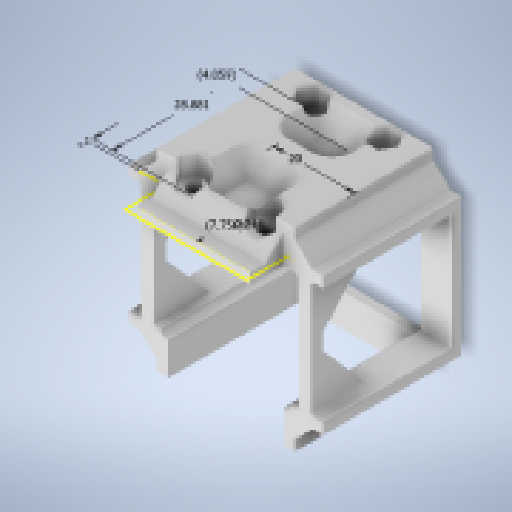
# Autodesk Inventor part: 56-spiralxy-groove-FocusToCubeAdapter
Saved by Autodesk Inventor 2024.1 (Build 281209000, 209)
## iProperties
Created: 2023-11-15
Part Number: 56-spiralxy-groove-FocusToCubeAdapter
Material: Generisch
Document SubType Name: Modeling
Designer: buchmannmartin
Density: 1 g/cm^3
Appearance: Vorgabe
Author: buchmannmartin
Autodesk Inventor part; units mm, degrees
ref_plane "YZ Plane" through (0, 0, 0) normal (1, 0, 0) x (0, 1, 0)
ref_plane "XZ Plane" through (0, 0, 0) normal (0, 1, 0) x (-1, 0, 0)
ref_plane "XY Plane" through (0, 0, 0) normal (0, 0, 1) x (1, 0, 0)
sketch "Skizze1" plane through (0, 0, 0) normal (0, 0, 1) x (1, 0, 0)
  line L0 (17.02, 23.9) -> (17.02, 21.2698) construction
  line L1 (17.02, 21.2698) -> (21.2698, 17.02) construction
  line L2 (21.2698, 17.02) -> (23.9, 17.02) construction
  line L3 (-23.9, 17.02) -> (-21.2698, 17.02) construction
  line L4 (-21.2698, 17.02) -> (-17.02, 21.2698) construction
  line L5 (-17.02, 21.2698) -> (-17.02, 23.9) construction
  line L6 (-17.02, -23.9) -> (-17.02, -21.2698) construction
  line L7 (-17.02, -21.2698) -> (-21.2698, -17.02) construction
  line L8 (-21.2698, -17.02) -> (-23.9, -17.02) construction
  line L9 (23.9, -17.02) -> (21.2698, -17.02) construction
  line L10 (21.2698, -17.02) -> (17.02, -21.2698) construction
  line L11 (17.02, -21.2698) -> (17.02, -23.9) construction
  line L12 (-14.5, 14.25) -> (14.5, 14.25)
  line L13 (16, 12.75) -> (16, -14.25)
  line L14 (14.5, -15.75) -> (-14.5, -15.75)
  line L15 (-16, -14.25) -> (-16, 12.75)
  line L16 (17.02, 23.9) -> (-17.02, 23.9) construction
  line L17 (-23.9, 17.02) -> (-23.9, -17.02) construction
  line L18 (23.9, -17.02) -> (23.9, 17.02) construction
  line L19 (17.02, -23.9) -> (-17.02, -23.9) construction
  line L20 (-16.92, 23.8) -> (-16.92, 21.2284)
  line L21 (-16.92, 21.2284) -> (-21.2284, 16.92)
  line L22 (-21.2284, 16.92) -> (-23.8, 16.92)
  line L23 (-23.8, 16.92) -> (-23.8, -16.92)
  line L24 (-23.8, -16.92) -> (-21.2284, -16.92)
  line L25 (-21.2284, -16.92) -> (-16.92, -21.2284)
  line L26 (-16.92, -21.2284) -> (-16.92, -23.8)
  line L27 (-16.92, -23.8) -> (16.92, -23.8)
  line L28 (16.92, -23.8) -> (16.92, -21.2284)
  line L29 (16.92, -21.2284) -> (21.2284, -16.92)
  line L30 (21.2284, -16.92) -> (23.8, -16.92)
  line L31 (23.8, -16.92) -> (23.8, 16.92)
  line L32 (23.8, 16.92) -> (21.2284, 16.92)
  line L33 (21.2284, 16.92) -> (16.92, 21.2284)
  line L34 (16.92, 21.2284) -> (16.92, 23.8)
  line L35 (16.92, 23.8) -> (-16.92, 23.8)
  arc A0 (16, 12.75) -> (14.5, 14.25) centre (14.5, 12.75) ccw
  arc A1 (14.5, -15.75) -> (16, -14.25) centre (14.5, -14.25) ccw
  arc A2 (-16, -14.25) -> (-14.5, -15.75) centre (-14.5, -14.25) ccw
  arc A3 (-14.5, 14.25) -> (-16, 12.75) centre (-14.5, 12.75) ccw
  point P0 (0, 0)
  point P1 (0, -15.75)
  dimension "d2" = 360
  dimension "d4" = 54.15
  dimension "d5" = 34.04
  dimension "d6" = 47.8
  dimension "d10" = 0.1
  dimension "d11" = 1.5
  dimension "d15" = 29
  dimension "d16" = 30
  dimension "d19" = 14.25
  constraints: 72 end point, 8 perpendicular, 8 point on circle, 8 tangent, 4 centre point, 4 parallel, 3 equal radius, 2 collinear, 2 horizontal, 2 vertical alignment, 1 horizontal alignment, 1 midpoint, 1 vertical, 44 other
  measures "d4" distance between parallel lines of L10 L4
  measures "d5" distance between parallel lines of L11 L6
  measures "d6" distance of L6.start L5.end
  measures "d10" distance between parallel lines of L35 L16
  measures "d11" radius of A0
  measures "d15" distance of A2.centre A1.centre
  measures "d16" distance between parallel lines of L12 L14
  measures "d19" distance from line of point (0, 0) L12
extrude "Extrusion1" add sketch "Skizze1" along normal blind 33.94
sketch "Skizze2" plane through (0, 0, 0) normal (1, 0, 0) x (0, 1, 0)
  line L0 (-15.75, 0) -> (-15.75, 33.94) construction
  line L1 (-15.75, 33.94) -> (-15.75, 38.29) construction
  line L2 (-15.75, 38.29) -> (-18.3, 38.29) construction
  line L3 (-18.3, 38.29) -> (-22.65, 33.94)
  line L4 (-22.65, 33.94) -> (-15.75, 33.94)
  line L5 (-15.75, 33.94) -> (-15.75, 41.94)
  line L6 (-15.75, 41.94) -> (-18.3, 41.94)
  line L7 (-18.3, 41.94) -> (-18.3, 38.29)
  line L8 (-0.75, 41.3732) -> (-0.75, 30.0346) construction
  line L9 (16.8, 38.29) -> (21.15, 33.94)
  line L10 (21.15, 33.94) -> (14.25, 33.94)
  line L11 (14.25, 33.94) -> (14.25, 41.94)
  line L12 (14.25, 41.94) -> (16.8, 41.94)
  line L13 (16.8, 41.94) -> (16.8, 38.29)
  line L14 (14.25, 0) -> (14.25, 33.94) construction
  line L15 (-23.8, 0) -> (-23.8, 33.94) construction
  line L16 (23.8, 0) -> (23.8, 33.94) construction
  point P0 (0, 0)
  dimension "d21" = 45
  dimension "d23" = 8
  dimension "d26" = 16.8
  dimension "d28" = 1.15
  dimension "d29" = 2.65
  constraints: 26 end point, 5 symmetric about line, 3 perpendicular, 2 vertical, 1 collinear, 1 horizontal, 1 point on line
  measures "d21" angle of L4 L3
  measures "d23" distance between parallel lines of L4 L6
  measures "d26" distance from line of L13 point (0, 0)
  measures "d28" distance from line of L3.end L15
  measures "d29" distance from line of L9.end L16
extrude "Extrusion2" add sketch "Skizze2" along normal mid plane 28 contours L9 L10 L11 L12 L13
sketch "Skizze3" plane through (-16.92, 16.8, 0) normal (0, 1, 0) x (1, 0, 0)
  line L0 (33.84, 0) -> (0, 0) construction
  line L1 (0, 0) -> (0, -33.94) construction
  line L2 (33.84, -33.94) -> (0, -33.94) construction
  line L3 (33.84, 0) -> (33.84, -33.94) construction
  line L4 (2.92, -41.94) -> (30.92, -41.94) construction
  line L5 (6.92, -14.184) -> (26.92, -14.184) construction
  line L6 (26.92, -14.184) -> (26.92, -34.184) construction
  line L7 (26.92, -34.184) -> (6.92, -34.184) construction
  line L8 (6.92, -34.184) -> (6.92, -14.184) construction
  circle A0 centre (25.67, -6.47) radius 1.7 projected
  circle A1 centre (8.17, -35.47) radius 1.7 projected
  circle A2 centre (25.67, -35.47) radius 1.7 projected
  circle A3 centre (8.17, -6.47) radius 1.7 projected
  line L9 (1.92, 2.03) -> (31.92, 2.03) projected
  line L10 (1.92, -43.97) -> (1.92, 2.03) projected
  line L11 (31.92, -43.97) -> (1.92, -43.97) projected
  line L12 (31.92, 2.03) -> (31.92, -43.97) projected
  line L13 (25.67, -32.94) -> (8.17, -32.94)
  line L14 (8.17, -32.94) -> (8.17, -4.0594)
  line L15 (8.17, -4.0594) -> (25.67, -4.0594)
  line L16 (25.67, -4.0594) -> (25.67, -32.94)
  line L17 (-4.3084, -33.94) -> (0, -33.94) projected
  point P0 (16.92, 0)
  point P1 (16.92, -14.184)
  point P2 (16.92, 0)
  point P3 (16.92, -4.0594)
  dimension "d30" = 20
  dimension "d31" = 7.756
  dimension "d32" = 0.244
  dimension "d77" = 1
  dimension "d78" = 28.8806
  dimension "d79" = 4.0594
  constraints: 16 end point, 4 parallel, 3 midpoint, 3 perpendicular, 2 horizontal
  measures "d30" distance of L5.start L5.end
  measures "d31" distance between parallel lines of L7 L4
  measures "d32" distance between parallel lines of L2 L7
  measures "d77" distance between parallel lines of L17 L13
  measures "d78" distance from line of point (16.92, -4.059) L13
  measures "d79" distance from line of L15 L0.end
hole "Bohrung2" at (8.75, 16.8, 4.0594) at (-8.75, 16.8, 4.0594) at (-8.75, 16.8, 32.94) at (8.75, 16.8, 32.94) direction (0, -1, 0) diameter 3.4 end through all start extended yes clearance for "Inbusschraube ISO 4762" size "M3" standard "ISO"
ref_plane "Arbeitsebene1" through (0, 0, 2.1) normal (0, 0, -1) x (-1, 0, 0)
sketch "Skizze4" plane through (0, 0, 33.94) normal (0, 0, 1) x (1, 0, 0)
  line L0 (14, 21.15) -> (14, 14.25) construction
  line L1 (14, 14.25) -> (14.5, 14.25) construction
  arc A0 (16, 12.75) -> (14.5, 14.25) centre (14.5, 12.75) ccw construction
  line L2 (16, 12.75) -> (16, -14.25) construction
  arc A1 (14.5, -15.75) -> (16, -14.25) centre (14.5, -14.25) ccw construction
  line L3 (14.5, -15.75) -> (10.1248, -15.75) construction
  arc A2 (-16, -14.25) -> (-14.5, -15.75) centre (-14.5, -14.25) ccw construction
  line L4 (-16, -14.25) -> (-16, 12.75) construction
  arc A3 (-14.5, 14.25) -> (-16, 12.75) centre (-14.5, 12.75) ccw construction
  line L5 (-14.5, 14.25) -> (-14, 14.25) construction
  line L6 (-14, 14.25) -> (-14, 21.15) construction
  line L7 (-14, 21.15) -> (-10.1248, 21.15) construction
  line L8 (-16.92, 21.2284) -> (-21.2284, 16.92) construction
  line L9 (-21.2284, 16.92) -> (-23.8, 16.92) construction
  line L10 (-23.8, 16.92) -> (-23.8, -16.92) construction
  line L11 (-23.8, -16.92) -> (-21.2284, -16.92) construction
  line L12 (-21.2284, -16.92) -> (-16.92, -21.2284) construction
  line L13 (-16.92, -21.2284) -> (-16.92, -23.8) construction
  line L14 (-16.92, -23.8) -> (-10.1248, -23.8) construction
  line L15 (16.92, -23.8) -> (16.92, -21.2284) construction
  line L16 (16.92, -21.2284) -> (21.2284, -16.92) construction
  line L17 (21.2284, -16.92) -> (23.8, -16.92) construction
  line L18 (23.8, -16.92) -> (23.8, 16.92) construction
  line L19 (23.8, 16.92) -> (21.2284, 16.92) construction
  line L20 (21.2284, 16.92) -> (16.92, 21.2284) construction
  line L21 (16.92, 21.2284) -> (16.92, 23.8) construction
  line L22 (16.92, 23.8) -> (10.1248, 23.8) construction
  line L23 (-16.92, 23.8) -> (-16.92, 21.2284) construction
  line L24 (-23.8, -14.25) -> (23.8, -14.25)
  line L25 (23.8, -14.25) -> (23.8, 14.25)
  line L26 (23.8, 14.25) -> (-23.8, 14.25)
  line L27 (-23.8, 14.25) -> (-23.8, -14.25)
  line L28 (-14.25, -23.8) -> (14.25, -23.8)
  line L29 (14.25, -23.8) -> (14.25, -14.25)
  line L30 (14.25, -14.25) -> (-14.25, -14.25)
  line L31 (-14.25, -14.25) -> (-14.25, -23.8)
  line L32 (7.3752, 21.15) -> (7.3752, 23.8) projected
  line L33 (7.3752, 23.8) -> (-7.3752, 23.8) projected
  line L34 (-7.3752, 23.8) -> (-7.3752, 21.15) projected
  line L35 (-7.3752, 21.15) -> (7.3752, 21.15) projected
  line L36 (7.3752, -23.8) -> (7.3752, -15.75) projected
  line L37 (7.3752, -15.75) -> (-7.3752, -15.75) projected
  line L38 (-7.3752, -15.75) -> (-7.3752, -23.8) projected
  line L39 (-7.3752, -23.8) -> (7.3752, -23.8) projected
  line L40 (-10.1248, 21.15) -> (-10.1248, 23.8) projected
  line L41 (-10.1248, 23.8) -> (-16.92, 23.8) projected
  line L42 (-10.1248, -23.8) -> (-10.1248, -15.75) projected
  line L43 (-10.1248, -15.75) -> (-14.5, -15.75) projected
  line L44 (10.1248, 23.8) -> (10.1248, 21.15) projected
  line L45 (10.1248, 21.15) -> (14, 21.15) projected
  line L46 (10.1248, -15.75) -> (10.1248, -23.8) projected
  line L47 (10.1248, -23.8) -> (16.92, -23.8) projected
  point P0 (0, 0)
  point P1 (0, -14.25)
  point P2 (0, -14.25)
  point P3 (-23.8, 0)
  point P4 (-14.25, 14.25)
  constraints: 16 end point, 5 midpoint, 4 parallel, 3 perpendicular, 2 horizontal, 2 point on line, 1 coincident, 1 collinear, 1 vertical alignment
extrude "Extrusion3" cut sketch "Skizze4" against normal up to surface (31.84 mm away) contours L27 L26 L25 L24 | L24 L29 L28 L36 L37 L38 L42 L43 L31 | L43 L42 L28 L31 | L28 L38 L37 L36
sketch "Skizze5" plane through (0, 0, 0) normal (1, 0, 0) x (0, 1, 0)
  line L0 (-14.25, 2.1) -> (-14.25, 33.94) construction
  line L1 (14.25, 33.94) -> (14.25, 2.1) construction
  line L2 (-14.25, 33.94) -> (14.25, 33.94)
  line L3 (14.25, 33.94) -> (14.25, 20.1)
  line L4 (14.25, 20.1) -> (2, 30.94)
  line L5 (2, 30.94) -> (-2, 30.94)
  line L6 (-2, 30.94) -> (-14.25, 20.1)
  line L7 (-14.25, 20.1) -> (-14.25, 33.94)
  point P0 (0, 0)
  point P1 (0, 30.94)
  point P2 (0, 33.94)
  dimension "d53" = 4
  dimension "d54" = 3
  dimension "d55" = 18
  dimension "d56" = 48.495
  constraints: 12 end point, 2 collinear, 2 midpoint, 1 horizontal, 1 horizontal alignment, 1 parallel, 1 perpendicular, 1 vertical alignment
  measures "d53" distance of L4.end L5.end
  measures "d54" distance between parallel lines of L2 L5
  measures "d55" distance of L1.end L3.end
  measures "d56" angle of L1 L4
extrude "Extrusion4" add sketch "Skizze5" against normal blind 6 from surface at 23.8
extrude "Extrusion5" cut sketch "Skizze5" against normal blind 3 from surface at 23.8
pattern_circular "Runde Anordnung1" count 2 over 360 about axis through (0, 0, -10) along (0, 0, -1) of "Extrusion4", "Extrusion5"
fillet "Rundung1" radius 1 4 edges at (20.8, -14.25, 27.02) (17.8, -14.25, 27.02) (20.8, 14.25, 27.02) (17.8, 14.25, 27.02)
sketch "Skizze6" plane through (-16.92, 23.8, 0) normal (0, 1, 0) x (1, 0, 0)
  arc A0 (25.4144, -37.1507) -> (27.1756, -36.2593) centre (26.92, -37.94) ccw construction
  circle A1 centre (6.92, -17.94) radius 1.7 construction
  line L0 (19.8489, -35.8689) -> (13.9911, -35.8689)
  line L1 (8.9911, -30.8689) -> (8.9911, -25.0111)
  line L2 (13.9911, -20.0111) -> (19.8489, -20.0111)
  line L3 (24.8489, -25.0111) -> (24.8489, -30.8689)
  arc A2 (19.8489, -35.8689) -> (24.8489, -30.8689) centre (19.8489, -30.8689) ccw
  arc A3 (24.8489, -25.0111) -> (19.8489, -20.0111) centre (19.8489, -25.0111) ccw
  arc A4 (13.9911, -20.0111) -> (8.9911, -25.0111) centre (13.9911, -25.0111) ccw
  line L4 (32.92, -2.1) -> (40.72, -2.1) construction
  arc A5 (8.9911, -30.8689) -> (13.9911, -35.8689) centre (13.9911, -30.8689) ccw
  line L5 (13.9911, -30.8689) -> (19.8489, -25.0111) construction
  line L6 (19.8489, -30.8689) -> (13.9911, -25.0111) construction
  circle A6 centre (6.92, -17.94) radius 4 construction
  line L7 (26.92, -37.94) -> (6.92, -17.94) construction
  line L8 (6.92, -17.94) -> (26.92, -17.94) construction
  line L9 (16.92, 0) -> (16.92, -17.94) construction
  line L10 (19.8489, -15.8689) -> (13.9911, -15.8689)
  line L11 (8.9911, -10.8689) -> (8.9911, -7.1)
  line L12 (13.9911, -2.1) -> (19.8489, -2.1)
  line L13 (24.8489, -7.1) -> (24.8489, -10.8689)
  arc A7 (19.8489, -15.8689) -> (24.8489, -10.8689) centre (19.8489, -10.8689) ccw
  arc A8 (24.8489, -7.1) -> (19.8489, -2.1) centre (19.8489, -7.1) ccw
  arc A9 (13.9911, -2.1) -> (8.9911, -7.1) centre (13.9911, -7.1) ccw
  arc A10 (8.9911, -10.8689) -> (13.9911, -15.8689) centre (13.9911, -10.8689) ccw
  line L14 (19.8489, -10.8689) -> (13.9911, -7.1) construction
  point P0 (16.92, -27.94)
  point P1 (16.92, -8.9845)
  dimension "d65" = 5
  dimension "d67" = 1
  constraints: 28 end point, 16 point on circle, 16 tangent, 8 centre point, 7 equal radius, 6 midpoint, 4 parallel, 3 horizontal, 3 perpendicular, 2 collinear, 1 point on line, 1 vertical alignment, 1 other
  measures "d65" radius of A2
extrude "Extrusion6" cut sketch "Skizze6" against normal blind 5 draft -40
chamfer "Fasen1" [suppressed]
chamfer "Fasen2" [suppressed]
sketch "Skizze7" plane through (-2.9289, 23.8, 20.0111) normal (0, 1, 0) x (1, 0, 0)
  line L0 (0, 17.9111) -> (5.8579, 17.9111) projected
  arc A0 (9.9949, 15.719) -> (5.8579, 17.9111) centre (5.8579, 12.9111) ccw projected
  line L1 (10.8579, 12.9111) -> (10.8579, 9.1421) projected
  arc A1 (5.8579, 4.1421) -> (10.8579, 9.1421) centre (5.8579, 9.1421) ccw projected
  line L2 (5.8579, 4.1421) -> (0, 4.1421) projected
  arc A2 (-5, 9.1421) -> (0, 4.1421) centre (0, 9.1421) ccw projected
  line L3 (-5, 9.1421) -> (-5, 12.9111) projected
  arc A3 (-4.6681, 14.7024) -> (-5, 12.9111) centre (0, 12.9111) ccw projected
  arc A4 (-4.1371, 15.719) -> (-4.6681, 14.7024) centre (-5.8211, 15.9517) ccw projected
  arc A5 (10.5259, 14.7024) -> (9.9949, 15.719) centre (11.6789, 15.9517) ccw projected
  arc A6 (-4.9635, -11.4611) -> (-7.1958, -13.9289) centre (-5.8211, -12.9289) ccw projected
  line L4 (-5, -10.8579) -> (-5, -5) projected
  arc A7 (0, 0) -> (-5, -5) centre (0, -5) ccw projected
  line L5 (0, 0) -> (5.8579, 0) projected
  arc A8 (10.8579, -5) -> (5.8579, 0) centre (5.8579, -5) ccw projected
  line L6 (10.8579, -5) -> (10.8579, -10.8579) projected
  arc A9 (10.0869, -13.5252) -> (10.3042, -13.9289) centre (11.6789, -12.9289) ccw projected
  line L7 (19.8489, 20.0111) -> (19.8489, -13.9289) projected
  line L8 (-13.9911, 20.0111) -> (-13.9911, -13.9289) projected
  line L9 (12.0918, -13.6441) -> (11.2661, -13.6441)
  line L10 (11.2661, -13.6441) -> (10.8532, -12.9289)
  line L11 (10.8532, -12.9289) -> (11.2661, -12.2138)
  line L12 (11.2661, -12.2138) -> (12.0918, -12.2138)
  line L13 (12.0918, -12.2138) -> (12.5047, -12.9289)
  line L14 (12.5047, -12.9289) -> (12.0918, -13.6441)
  circle A10 centre (-5.8211, -12.9289) radius 1.7 projected
  line L15 (-4.0024, -9.7789) -> (-2.1838, -12.9289)
  line L16 (-2.1838, -12.9289) -> (-4.0024, -16.0789)
  line L17 (-4.0024, -16.0789) -> (-7.6397, -16.0789)
  line L18 (-7.6397, -16.0789) -> (-9.4584, -12.9289)
  line L19 (-9.4584, -12.9289) -> (-7.6397, -9.7789)
  line L20 (-7.6397, -9.7789) -> (-4.0024, -9.7789)
  line L21 (9.8603, 19.1017) -> (13.4976, 19.1017)
  line L22 (13.4976, 19.1017) -> (15.3162, 15.9517)
  line L23 (15.3162, 15.9517) -> (13.4976, 12.8017)
  line L24 (13.4976, 12.8017) -> (9.8603, 12.8017)
  line L25 (9.8603, 12.8017) -> (8.0416, 15.9517)
  line L26 (8.0416, 15.9517) -> (9.8603, 19.1017)
  line L27 (19.8489, -13.4289) -> (12.1637, -13.4289) projected
  line L28 (-6.3058, -13.4289) -> (-13.9911, -13.4289) projected
  line L29 (11.1593, -9.0289) -> (14.7966, -10.5289)
  line L30 (14.7966, -10.5289) -> (15.3162, -14.4289)
  line L31 (15.3162, -14.4289) -> (12.1985, -16.8289)
  line L32 (12.1985, -16.8289) -> (8.5612, -15.3289)
  line L33 (8.5612, -15.3289) -> (8.0416, -11.4289)
  line L34 (8.0416, -11.4289) -> (11.1593, -9.0289)
  line L35 (-7.6397, 19.1017) -> (-4.0024, 19.1017)
  line L36 (-4.0024, 19.1017) -> (-2.1838, 15.9517)
  line L37 (-2.1838, 15.9517) -> (-4.0024, 12.8017)
  line L38 (-4.0024, 12.8017) -> (-7.6397, 12.8017)
  line L39 (-7.6397, 12.8017) -> (-9.4584, 15.9517)
  line L40 (-9.4584, 15.9517) -> (-7.6397, 19.1017)
  arc A11 (-5, -10.8579) -> (-4.9635, -11.4611) centre (0, -10.8579) ccw projected
  arc A12 (10.8213, -11.4611) -> (10.8579, -10.8579) centre (5.8579, -10.8579) ccw projected
  arc A13 (13.0537, -13.9289) -> (10.8213, -11.4611) centre (11.6789, -12.9289) ccw projected
  line L41 (19.8489, -13.9289) -> (13.0537, -13.9289) projected
  line L42 (19.8489, 20.0111) -> (-13.9911, 20.0111) projected
  line L43 (-7.1958, -13.9289) -> (-13.9911, -13.9289) projected
  arc A14 (0, 17.9111) -> (-4.1371, 15.719) centre (0, 12.9111) ccw projected
  arc A15 (10.8579, 12.9111) -> (10.5259, 14.7024) centre (5.8579, 12.9111) ccw projected
  arc A16 (-4.2291, -13.5252) -> (-3.9457, -13.9289) centre (0, -10.8579) ccw projected
  arc A17 (-4.4463, -13.9289) -> (-4.2291, -13.5252) centre (-5.8211, -12.9289) ccw projected
  line L44 (-3.9457, -13.9289) -> (-4.4463, -13.9289) projected
  arc A18 (9.8036, -13.9289) -> (10.0869, -13.5252) centre (5.8579, -10.8579) ccw projected
  line L45 (10.3042, -13.9289) -> (9.8036, -13.9289) projected
  point P0 (-5.9745, -13.122)
  point P1 (-5, -9.9404)
  point P2 (11.6789, 19.1017)
  point P3 (11.6789, 12.8017)
  dimension "d80" = 6.3
  dimension "d81" = 6.3
  constraints: 60 end point, 5 coincident, 2 midpoint, 2 parallel, 1 collinear, 66 other
  measures "d80" distance between parallel lines of L20 L17
  measures "d81" distance of point (11.679, 19.102) point (11.679, 12.802)
extrude "Extrusion7" cut sketch "Skizze7" against normal blind 5 contours A14 A4 A3 L3 L38 L39 L40 L35 L36 | L36 L37 L38 L3 A3 A4 A14 | L26 L21 L22 L23 L24 L1 A15 A5 A0 | A0 A5 A15 L1 L24 L25 L26 | A10 A6 | A11 L4 L20 L15 L16 L17 L18 L43 A10 L44 A16 | A6 L28 L18 L19 L20 L4 A11 | A6 L43 L18 L28 | A16 L44 A10 | L30 L41 A13 L27 | L27 A13 A12 L6 L34 L29 L30 | L6 A12 A13 L41 L30 L31 L32 L33 L34 | A9 L45 A18 | L9 L10 L11 L12 L13 L14
